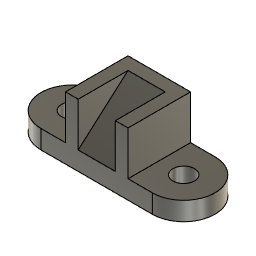
A2 (Autodesk Fusion 360 design; units mm, degrees)
Autodesk Fusion 360 part; units mm, degrees
sketch "Sketch1" plane through (0, 0, 0) normal (0, 0, 1) x (1, 0, 0)
  line L0 (57, 32) -> (-57, 32)
  line L1 (-57, -32) -> (57, -32)
  circle A0 centre (57, 0) radius 11
  circle A1 centre (-57, 0) radius 11
  arc A2 (57, -32) -> (57, 32) centre (57, 0) ccw
  arc A3 (-57, 32) -> (-57, -32) centre (-57, 0) ccw
  dimension "d1" = 114
  dimension "d2" = 64
  dimension "d3" = 32
  dimension "d4" = 32
  constraint horizontal L0
  constraint parallel L0 L1
  measures "d1" distance of L1.start L1.end
  measures "d2" distance of L0.end L1.start
  measures "d3" radius of A2
  measures "d4" radius of A3
extrude "Extrude1" add sketch "Sketch1" along normal blind 19
sketch "Sketch2" plane through (0, 0, 0) normal (0, 1, 0) x (1, 0, 0)
  line L0 (-32, -19) -> (-19, -19)
  line L1 (-19, -19) -> (-19, -64)
  line L2 (-19, -64) -> (-32, -64)
  line L3 (-32, -64) -> (-32, -19)
  line L4 (-57, 0) -> (-57, -19)
  dimension "d9" = 13
  dimension "d10" = 45
  dimension "d11" = 25
  constraint horizontal L0
  constraint vertical L1
  constraint horizontal L2
  constraint vertical L3
  measures "d9" distance of L0.start L0.end
  measures "d10" distance of L0.start L2.end
  measures "d11" distance of L3 L4
extrude "Extrude2" add sketch "Sketch2" along normal mid plane 64
sketch "Sketch3" plane through (0, 0, 0) normal (0, 1, 0) x (1, 0, 0)
  line L0 (32, -19) -> (19, -19)
  line L1 (19, -19) -> (19, -64)
  line L2 (19, -64) -> (32, -64)
  line L3 (32, -64) -> (32, -19)
  line L4 (57, 0) -> (57, -19)
  dimension "d14" = 13
  dimension "d15" = 45
  dimension "d16" = 25
  constraint horizontal L0
  constraint vertical L1
  constraint horizontal L2
  constraint vertical L3
  measures "d14" distance of L0.start L0.end
  measures "d15" distance of L0.start L2.end
  measures "d16" distance of L3 L4
extrude "Extrude3" add sketch "Sketch3" along normal mid plane 64
sketch "Sketch5" plane through (0, 32, 0) normal (0, 1, 0) x (-1, 0, 0)
  line L0 (-57, 0) -> (57, 0)
  line L1 (57, 0) -> (57, 19)
  line L2 (57, 19) -> (32, 19)
  line L3 (32, 19) -> (32, 64)
  line L4 (32, 64) -> (19, 64)
  line L5 (19, 64) -> (19, 19)
  line L6 (19, 19) -> (-19, 19)
  line L7 (-19, 19) -> (-19, 64)
  line L8 (-19, 64) -> (-32, 64)
  line L9 (-32, 64) -> (-32, 19)
  line L10 (-32, 19) -> (-57, 19)
  line L11 (-57, 19) -> (-57, 0)
  line L12 (-19, 19) -> (19, 19)
  line L13 (19, 19) -> (19, 64)
  line L14 (19, 64) -> (-19, 64)
  line L15 (-19, 64) -> (-19, 19)
  constraint horizontal L12
  constraint vertical L13
  constraint horizontal L14
  constraint vertical L15
  constraint coincident L4.end L5.start
  constraint coincident L6.end L7.start
extrude "Extrude4" add sketch "Sketch5" against normal blind 13 contours L5 L6 L7 L12 L13 L14 L15
sketch "Sketch6" plane through (-19, 0, 0) normal (1, 0, 0) x (0, 1, 0)
  line L0 (19, 19) -> (19, 64)
  line L1 (19, 64) -> (-32, 64)
  line L2 (-32, 64) -> (-32, 19)
  line L3 (-32, 19) -> (19, 19)
  line L4 (19, 64) -> (-32, 19)
  line L5 (19, 19) -> (19, 64)
  line L6 (-32, 19) -> (19, 19)
  constraint coincident L0.end L1.start
  constraint coincident L2.end L3.start
  constraint coincident L0.start L3.end
extrude "Extrude5" add sketch "Sketch6" along normal blind 38 contours L0 L3 L4 L5 L6
